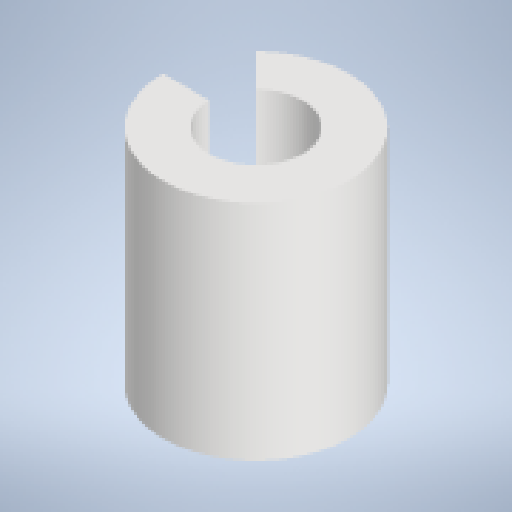
# Autodesk Inventor part: Piston Spacer
Saved by Autodesk Inventor 2023 (Build 270158000, 158)
## iProperties
Created: 2023-03-02
Part Number: Piston Spacer
Material: Generic
Document SubType Name: Modeling
Designer: Gabriel - T3 CAD
Density: 1 g/cm^3
Appearance: Default
Author: Gabriel - T3 CAD
Autodesk Inventor part; units mm, degrees
ref_plane "YZ Plane" through (0, 0, 0) normal (1, 0, 0) x (0, 1, 0)
ref_plane "XZ Plane" through (0, 0, 0) normal (0, 1, 0) x (-1, 0, 0)
ref_plane "XY Plane" through (0, 0, 0) normal (0, 0, 1) x (1, 0, 0)
sketch "Sketch1" plane through (0, 0, 0) normal (0, 1, 0) x (-1, 0, 0)
  circle A0 centre (0, 0) radius 3.175
  circle A1 centre (0, 0) radius 6.35
  line L0 (6.35, 0) -> (0, 0)
  line L1 (0, 0) -> (4.4901, -4.4901)
  point P0 (2.2451, -2.2451)
  point P1 (3.175, 0)
  dimension "d0" = 6.35
  dimension "d1" = 12.7
  dimension "d2" = 45
  constraints: 4 coincident, 4 end point, 2 centre point, 2 point on circle, 1 horizontal
  measures "d0" diameter of A0
  measures "d1" diameter of A1
  measures "d2" angle of L1 L0
extrude "Extrusion1" add sketch "Sketch1" along normal blind 15.24 contours A0 L1 A1 L0 picked at (-0.4127, 5.2358)
body "Solid1"
